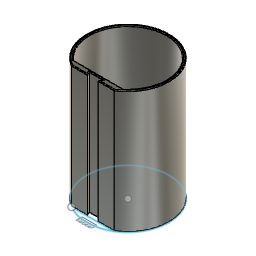
Cookie part of jar v2 (Autodesk Fusion 360 design; units mm, degrees)
Autodesk Fusion 360 part; units mm, degrees
note: some values were not read from the file. Set by a fixed rule: which sketch regions a step uses.
sketch "Sketch1" plane through (0, 0, 0) normal (0, 0, 1) x (1, 0, 0)
  line L0 (0, 5) -> (10, 5)
  line L1 (0, 5) -> (-10, 5)
  line L2 (-7.5, 0) -> (-10, 5)
  line L3 (10, 5) -> (7.5, 0)
  line L4 (-7.5, 0) -> (-30.375, 0)
  line L5 (7.5, 0) -> (30.375, 0)
  line L6 (0, 0) -> (0, 50)
  circle A0 centre (0, 50) radius 58.5033
  constraint horizontal L4
  constraint horizontal L5
  constraint coincident L6.start origin
  constraint perpendicular L0 L6
  constraint coincident L6.end A0.centre
  constraint coincident L4.end A0
extrude "Extrude1" add sketch "Sketch1" along normal blind 174.5 contours L0 L1 L2 L3 L4 L5 A0 picked at (-15.3089, 35.3909)
sketch "Sketch2" plane through (0, 0, 174.5) normal (0, 0, 1) x (-1, 0, 0)
  line L0 (10, -5) -> (-10, -5)
  line L1 (-10, -5) -> (-7.5, 0)
  line L2 (-7.5, 0) -> (-30.375, 0)
  arc A0 (-30.375, 0) -> (30.375, 0) centre (0, -50) ccw
  line L3 (30.375, 0) -> (7.5, 0)
  line L4 (7.5, 0) -> (10, -5)
  circle A1 centre (0, -50) radius 55
  line L5 (0, -5) -> (0, -8)
  line L6 (0, -8) -> (-35.5106, -8)
  line L7 (0, -8) -> (35.5106, -8)
  dimension "d10" = 3
  constraint concentric A0 A1
  constraint midpoint L0 L5.start
  constraint perpendicular L0 L5
  constraint coincident A1 L6.end
  constraint perpendicular L5 L6
  constraint coincident A1 L7.end
  constraint perpendicular L5 L7
  measures "d10" distance of L5.start L5.end
extrude "Extrude2" cut sketch "Sketch2" against normal blind 170 contours A1 L6 L7
fillet "Fillet1" radius 1 1 faces at (25.2952, 4.3333, 174.5)
fillet "Fillet2" radius 1 1 faces at (-15.3089, 35.3909, 0)
sketch "Sketch3" plane through (0, 0, 0) normal (0, 0, 1) x (1, 0, 0)
  line L0 (-30, 0) -> (30, 0)
  circle A0 centre (0, 50) radius 58.3095
  constraint horizontal L0
  constraint coincident L0.end A0
